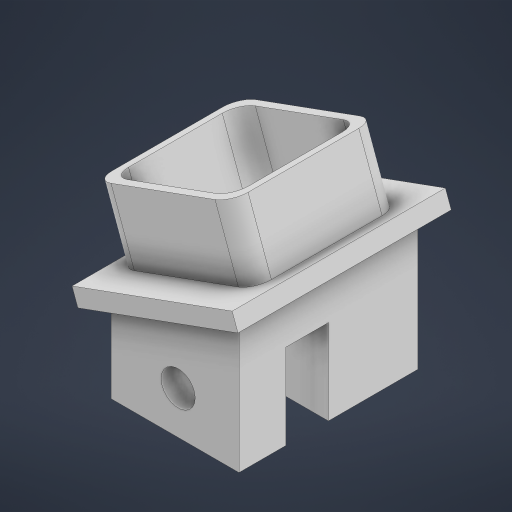
# Autodesk Inventor part: base_70
Saved by Autodesk Inventor 2024 (Build 280153000, 153)
## iProperties
Created: 2023-05-28
Part Number: base_70
Material: Типовые
Document SubType Name: Modeling
Designer: user
Density: 1 g/cm^3
Appearance: По умолчанию
Author: user
Autodesk Inventor part; units mm, degrees
ref_plane "YZ Plane" through (0, 0, 0) normal (1, 0, 0) x (0, 1, 0)
ref_plane "XZ Plane" through (0, 0, 0) normal (0, 1, 0) x (-1, 0, 0)
ref_plane "XY Plane" through (0, 0, 0) normal (0, 0, 1) x (1, 0, 0)
sketch "Эскиз1" plane through (0, 0, 0) normal (0, 0, 1) x (1, 0, 0)
  line L0 (7.5, -5) -> (7.5, 0) projected
  line L1 (5.0577, -5) -> (7.5, -5) projected
  line L2 (5.0577, -5) -> (-4.3392, -5) projected
  line L3 (-6.7815, -5) -> (-4.3392, -5) projected
  line L4 (-6.7815, -5) -> (-6.7815, 0) projected
  line L5 (-6.7815, 0) -> (-4.3392, 0) projected
  line L6 (5.0577, 0) -> (-4.3392, 0) projected
  line L7 (5.0577, 0) -> (7.5, 0) projected
  line L8 (7.5, -10.5) -> (-7.5, -10.5) projected
  line L9 (7.5, 0) -> (-6.7815, 0) projected
  line L10 (7.5, 10.5) -> (7.5, 0) projected
  line L11 (-7.5, 10.5) -> (7.5, 10.5) projected
  line L12 (-7.5, -10.5) -> (-7.5, 10.5) projected
  line L13 (7.5, -10.5) -> (-7.5, -10.5) projected
  line L14 (7.5, -5) -> (7.5, -10.5) projected
  line L15 (7.5, -5) -> (-6.7815, -5) projected
  line L16 (-6.7815, -5) -> (-6.7815, 0) projected
  point P0 (0, 0)
extrude "Выдавливание1" add sketch "Эскиз1" along normal blind 10 contours L14 L8 L12 L11 L10 L7 L6 L5 L4 L3 L2 L1
sketch "Эскиз2" plane through (-7.5, 10.5, 0) normal (0, 1, 0) x (1, 0, 0)
  circle A0 centre (7.8593, -5) radius 2 projected
  point P0 (7.5, 0)
extrude "Выдавливание2" cut sketch "Эскиз2" against normal through all
sketch "Эскиз3" plane through (-7.5, 10.5, 0) normal (0, 1, 0) x (1, 0, 0)
  line L0 (15, -10) -> (0, -10) projected
  line L1 (15, -10) -> (15, -15.4596)
  line L2 (15, -15.4596) -> (0, -10)
  point P0 (7.5, 0)
  dimension "d5" = 20
  constraints: 4 end point, 1 vertical
  measures "d5" angle of L0 L2
extrude "Выдавливание3" add sketch "Эскиз3" against normal up to surface (21 mm away)
sketch "Эскиз4" plane through (7.5, -10.5, 15.4596) normal (-0.3420201, 0, 0.9396926) x (0.9396926, 0, 0.3420201)
  line L0 (-15.9627, 0) -> (0, 0) projected
  line L1 (0, 21) -> (0, 0) projected
  line L2 (-15.9627, 21) -> (0, 21) projected
  line L3 (-15.9627, 21) -> (-15.9627, 0) projected
  line L4 (-17.9813, -2.0187) -> (2.0187, -2.0187)
  line L5 (2.0187, -2.0187) -> (2.0187, 23.0187)
  line L6 (2.0187, 23.0187) -> (-17.9813, 23.0187)
  line L7 (-17.9813, 23.0187) -> (-17.9813, -2.0187)
  point P0 (-12.3352, 10.5)
  dimension "d8" = 20
  constraints: 8 end point, 3 other
  measures "d8" distance of L4.start L4.end
extrude "Выдавливание4" add sketch "Эскиз4" along normal blind 2 contours L3 L2 L1 L0 | L7 L6 L5 L4
sketch "Эскиз5" plane through (6.816, -10.5, 17.3389) normal (-0.3420201, 0, 0.9396926) x (0.9396926, 0, 0.3420201)
  line L0 (0.5187, 19) -> (-16.4813, 19)
  line L1 (-16.4813, 19) -> (-16.4813, 2)
  line L2 (-16.4813, 2) -> (0.5187, 2)
  line L3 (0.5187, 2) -> (0.5187, 19)
  line L4 (2.0187, -2.0187) -> (2.0187, 23.0187) projected
  line L5 (-17.9813, -2.0187) -> (2.0187, -2.0187) projected
  line L6 (-0.4813, 18) -> (-15.4813, 18)
  line L7 (-15.4813, 18) -> (-15.4813, 3)
  line L8 (-15.4813, 3) -> (-0.4813, 3)
  line L9 (-0.4813, 3) -> (-0.4813, 18)
  point P0 (-12.3352, 10.5)
  point P1 (0.5187, 10.5)
  point P2 (2.0187, 10.5)
  point P3 (-7.9813, 2)
  point P4 (-7.9813, -2.0187)
  dimension "d11" = 17
  dimension "d12" = 1
  constraints: 16 end point, 4 midpoint, 4 parallel, 3 perpendicular, 1 horizontal, 1 horizontal alignment, 1 vertical alignment, 3 other
  measures "d11" distance of L0.end L1.end
  measures "d12" distance between parallel lines of L3 L9
extrude "Выдавливание5" add sketch "Эскиз5" along normal blind 8
fillet "Сопряжение1" radius 2 8 edges at (5.9353, -8.5, 21.2751) (5.9353, 8.5, 21.2751) (-10.0395, 8.5, 15.4608) (-10.0395, -8.5, 15.4608) (-9.0998, 7.5, 15.8028) (4.9956, 7.5, 20.9331) (-9.0998, -7.5, 15.8028) (4.9956, -7.5, 20.9331)
equation "\"degg\" = 70deg"
